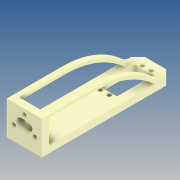
# Autodesk Inventor part: BONE_v3
Saved by Autodesk Inventor 2020.2 (Build 242310000, 310)
## iProperties
Created: 2020-03-23
Part Number: BONE_v3
Material: PLA plastic
Document SubType Name: Modeling
Designer: David
Mass: 66.3198 g
Surface Area: 224.05 cm^2
Volume: 53.0558 cm^3
Density: 1.25 g/cm^3
Appearance: PLA plastic
Author: David
Autodesk Inventor part; units mm, degrees
ref_plane "YZ Plane" through (0, 0, 0) normal (1, 0, 0) x (0, 1, 0)
ref_plane "XZ Plane" through (0, 0, 0) normal (0, 1, 0) x (-1, 0, 0)
ref_plane "XY Plane" through (0, 0, 0) normal (0, 0, 1) x (1, 0, 0)
sketch "Sketch1" plane through (0, 0, 0) normal (1, 0, 0) x (0, 1, 0)
  line L0 (0, 0) -> (8, 0)
  line L1 (8, 0) -> (8, 150)
  line L2 (8, 150) -> (0, 150)
  line L3 (0, 150) -> (0, 0)
  dimension "d0" = 150
  dimension "d1" = 8
  constraints: 8 end point, 2 parallel, 1 horizontal, 1 perpendicular
  measures "d0" distance of L0.end L1.end
  measures "d1" distance of L0.start L0.end
extrude "BODY1" add sketch "Sketch1" against normal blind 40
sketch "Sketch2" plane through (0, 8, 150) normal (0, 1, 0) x (1, 0, 0)
  line L0 (0, 0) -> (-40, 0)
  line L1 (-40, 0) -> (-40, 8)
  line L2 (-40, 8) -> (0, 8)
  line L3 (0, 8) -> (0, 0)
  dimension "d4" = 40
  dimension "d5" = 8
  constraints: 8 end point, 2 parallel, 1 horizontal, 1 perpendicular
  measures "d4" distance of L1.end L2.end
  measures "d5" distance of L0.end L1.end
extrude "BODY2" add sketch "Sketch2" along normal blind 30
sketch "Sketch3" plane through (-40, 8, 0) normal (0, 1, 0) x (1, 0, 0)
  line L0 (40, 0) -> (0, 0) construction
  line L1 (0, -142) -> (0, 0) construction
  circle A0 centre (15, -10) radius 2.25
  circle A1 centre (25, -10) radius 2.25
  circle A2 centre (15, -58) radius 2.25
  circle A3 centre (25, -58) radius 2.25
  line L2 (9, -13) -> (31, -13)
  line L3 (31, -13) -> (31, -55)
  line L4 (31, -55) -> (9, -55)
  line L5 (9, -55) -> (9, -13)
  dimension "d8" = 48
  dimension "d9" = 48
  dimension "d10" = 10
  dimension "d11" = 10
  dimension "d12" = 4.5
  dimension "d13" = 4.5
  dimension "d14" = 4.5
  dimension "d15" = 4.5
  dimension "d16" = 15
  dimension "d17" = 10
  dimension "d18" = 15
  dimension "d19" = 10
  dimension "d20" = 22
  dimension "d21" = 42
  dimension "d22" = 9
  dimension "d23" = 3
  constraints: 8 end point, 4 centre point, 2 parallel, 1 horizontal, 1 perpendicular
  measures "d8" distance of A1.centre A3.centre
  measures "d9" distance of A0.centre A2.centre
  measures "d10" distance of A2.centre A3.centre
  measures "d11" distance of A1.centre A0.centre
  measures "d12" diameter of A2
  measures "d13" diameter of A3
  measures "d14" diameter of A1
  measures "d15" diameter of A0
  measures "d16" distance from line of L1 A0.centre
  measures "d17" distance from line of L0 A0.centre
  measures "d18" distance from line of L1 A2.centre
  measures "d19" distance from line of L0 A1.centre
  measures "d20" distance between parallel lines of L3 L5
  measures "d21" distance between parallel lines of L2 L4
  measures "d22" distance between parallel lines of L1 L5
  measures "d23" distance from line of A2.centre L4
extrude "SERVO" cut sketch "Sketch3" against normal blind 8
sketch "Sketch4" plane through (0, 8, 142) normal (0, 0, -1) x (-1, 0, 0)
  line L0 (40, 0) -> (0, 0) construction
  line L1 (40, 0) -> (40, 30) construction
  line L2 (0, 30) -> (40, 30) construction
  line L3 (0, 0) -> (0, 30) construction
  line L4 (24, 19) -> (16, 19)
  line L5 (16, 19) -> (16, 9)
  line L6 (16, 9) -> (24, 9)
  line L7 (24, 9) -> (24, 19)
  arc A0 (24, 9) -> (24, 19) centre (24, 14) ccw
  arc A1 (16, 19) -> (16, 9) centre (16, 14) ccw
  circle A2 centre (20, 24) radius 2.25
  circle A3 centre (32, 8) radius 2.25
  circle A4 centre (8, 8) radius 2.25
  point P0 (0, -8)
  dimension "d26" = 11
  dimension "d28" = 8
  dimension "d29" = 10
  dimension "d30" = 16
  dimension "d32" = 4.5
  dimension "d33" = 4.5
  dimension "d34" = 4.5
  dimension "d35" = 20
  dimension "d36" = 8
  dimension "d37" = 8
  dimension "d39" = 6
  dimension "d40" = 8
  dimension "d41" = 8
  constraints: 8 end point, 5 centre point, 4 point on circle, 4 tangent, 2 parallel, 1 horizontal, 1 perpendicular
  measures "d26" distance between parallel lines of L2 L4
  measures "d28" distance between parallel lines of L5 L7
  measures "d29" distance of L6.end L4.start
  measures "d30" distance between parallel lines of L3 L5
  measures "d32" diameter of A3
  measures "d33" diameter of A4
  measures "d34" diameter of A2
  measures "d35" distance from line of L3 A2.centre
  measures "d36" distance from line of L3 A4.centre
  measures "d37" distance from line of L1 A3.centre
  measures "d39" distance from line of L2 A2.centre
  measures "d40" distance from line of A4.centre L0
  measures "d41" distance from line of L0 A3.centre
extrude "CONNECTION" cut sketch "Sketch4" against normal blind 8
chamfer "v3_servo_chamfer" distance 8 angle 45 2 edges at (0, 4, 0) (-40, 4, 0)
sketch "v3_ribs_sketch" plane through (0, 8, 142) normal (0, 0, -1) x (-1, 0, 0)
  line L0 (0, 30) -> (0, -8) construction
  line L1 (0, 30) -> (6, 30)
  line L2 (6, 30) -> (6, 27)
  line L3 (6, 27) -> (0, 27)
  line L4 (0, 27) -> (0, 30)
  line L5 (40, 30) -> (0, 30) construction
  line L6 (40, 30) -> (34, 30)
  line L7 (34, 30) -> (34, 27)
  line L8 (34, 27) -> (40, 27)
  line L9 (40, 27) -> (40, 30)
  dimension "d66" = 6
  dimension "d67" = 3
  dimension "d68" = 6
  dimension "d69" = 3
  constraints: 16 end point, 4 parallel, 2 horizontal, 2 perpendicular
  measures "d66" distance of L7.end L8.end
  measures "d67" distance of L6.end L7.end
  measures "d68" distance of L2.end L3.end
  measures "d69" distance of L1.end L2.end
sketch "Sketch8" plane through (-40, 8, 142) normal (0, 1, 0) x (1, 0, 0)
  line L0 (0, 0) -> (0, 134) construction
  line L1 (40, 134) -> (40, 0) construction
  line L2 (32, 142) -> (8, 142) construction
  line L3 (40, 127) -> (34, 127)
  line L4 (34, 127) -> (34, 121)
  line L5 (34, 121) -> (40, 121)
  line L6 (40, 121) -> (40, 127)
  line L7 (0, 127) -> (6, 127)
  line L8 (6, 127) -> (6, 121)
  line L9 (6, 121) -> (0, 121)
  line L10 (0, 121) -> (0, 127)
  point P0 (40, 142)
  dimension "d70" = 6
  dimension "d71" = 6
  dimension "d72" = 6
  dimension "d73" = 6
  dimension "d74" = 15
  dimension "d75" = 15
  constraints: 16 end point, 4 parallel, 2 horizontal, 2 perpendicular, 2 point on line
  measures "d70" distance of L7.start L7.end
  measures "d71" distance of L3.start L3.end
  measures "d72" distance of L3.end L4.end
  measures "d73" distance of L7.end L8.end
  measures "d74" distance between parallel lines of L2 L7
  measures "d75" distance between parallel lines of L2 L3
extrude "v3_ribs_extrusion1" add sketch "Sketch8" along normal blind 30
extrude "v3_ribs_extrusion2" add sketch "v3_ribs_sketch" along normal blind 122
chamfer "v3_ribs_chamfer1" distance 27 angle 45 2 edges at (-3, 35, 21) (-37, 35, 21)
fillet "v3_ribs_fillet1" radius 100 2 edges at (-3, 35, 47.9999) (-37, 35, 47.9999)
fillet "v3_ribs_fillet2" radius 100 2 edges at (-3, 38, 15) (-37, 38, 15)
fillet "v3_ribs_fillet3" radius 15 2 edges at (-3, 8, 15) (-37, 8, 15)
equation "\"d4\" = d2"
equation "\"d5\" = d1"
equation "\"d9\" = d8"
equation "\"d11\" = d10"
equation "\"d13\" = d12"
equation "\"d14\" = d12"
equation "\"d15\" = d12"
equation "\"d18\" = d16"
equation "\"d19\" = d17"
equation "\"d32\" = d12"
equation "\"d33\" = d12"
equation "\"d34\" = d12"
equation "\"d37\" = d36"
equation "\"d41\" = d40"
equation "\"d68\" = d66"
equation "\"d69\" = d67"
equation "\"d70\" = d72"
equation "\"d71\" = d72"
equation "\"d72\" = d66"
equation "\"d73\" = d66"
equation "\"d75\" = d74"
equation "\"d2\" = 40"
body "Solid1"
